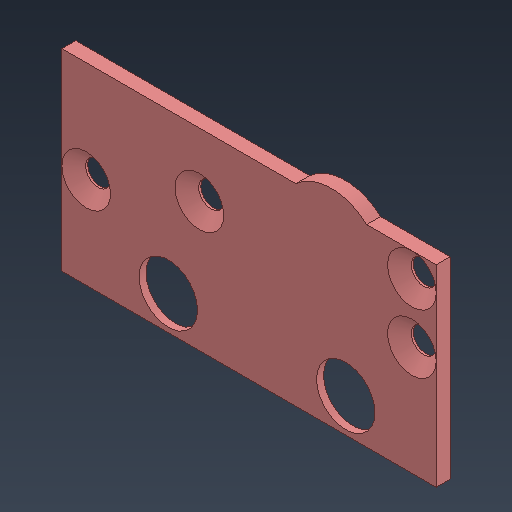
# Autodesk Inventor part: gearbox-holder-wall-right
Saved by Autodesk Inventor 2023 (Build 270158000, 158)
## iProperties
Created: 2025-04-06
Part Number: gearbox-holder-wall-right
Material: ABS Plastic
Document SubType Name: Modeling
Designer: szymo
Density: 1.06 g/cm^3
Appearance: Default(3)
Mass: 2.61652 g
Surface Area: 32.3606 cm^2
Volume: 2.46841 cm^3
Author: szymo
Autodesk Inventor part; units mm, degrees
ref_plane "YZ Plane" through (0, 0, 0) normal (1, 0, 0) x (0, 1, 0)
ref_plane "XZ Plane" through (0, 0, 0) normal (0, 1, 0) x (-1, 0, 0)
ref_plane "XY Plane" through (0, 0, 0) normal (0, 0, 1) x (1, 0, 0)
ref_plane "Work Plane7" through (-17.6, -15.9714, 1.1) normal (0, 0, 1) x (1, 0, 0)
ref_plane "Work Plane10" through (0, 0, 0.1) normal (0, 0, 1) x (1, 0, 0)
sketch "Sketch2" plane through (0, 0, 0.1) normal (0, 0, 1) x (1, 0, 0)
  line L0 (26.9, -14.8376) -> (26.9, 13.5936)
  line L1 (-26.9065, -14.8376) -> (26.9, -14.8376)
  circle A0 centre (-11.6, -9.9714) radius 6 projected
  circle A1 centre (13.9, -9.9714) radius 6 projected
  circle A2 centre (-11.6, -9.9714) radius 6.2
  circle A3 centre (13.9, -9.9714) radius 6.2
  arc A4 (-1.8466, -14.8376) -> (-21.3534, -14.8376) centre (-11.6, -9.9714) ccw
  line L2 (-1.8466, -14.8376) -> (4.1466, -14.8376)
  arc A5 (23.6534, -14.8376) -> (4.1466, -14.8376) centre (13.9, -9.9714) ccw
  line L3 (23.6534, -14.8376) -> (26.9, -14.8376)
  line L4 (26.9, -14.8376) -> (26.9, 12.8624)
  line L5 (26.9, 12.8624) -> (16.8986, 12.8624)
  arc A6 (16.8986, 12.8624) -> (6.7153, 12.8624) centre (11.8069, 7.2876) ccw
  line L6 (6.7153, 12.8624) -> (-26.9, 12.8624)
  line L7 (-26.9, 12.8624) -> (-26.9, -14.8376)
  line L8 (-26.9, -14.8376) -> (-21.3534, -14.8376)
  point P0 (0, 0)
  point P1 (-15.4418, -14.8376)
  point P2 (-7.7582, -14.8376)
  point P3 (10.0582, -14.8376)
  point P4 (17.7418, -14.8376)
  point P5 (-1.8466, -14.8376)
  point P6 (-15.1099, -14.8376)
  point P7 (-8.0901, -14.8376)
  point P8 (-26.9, -14.8376)
  point P9 (26.9, 12.8624)
  dimension "d2" = 0.2
  dimension "d3" = 0.2
  constraints: 18 end point, 6 point on circle, 5 centre point, 1 point on line
  measures "d2" radial gap between concentric circles of A0 A2
  measures "d3" radial gap between concentric circles of A1 A3
extrude "Extrusion2" add sketch "Sketch2" along normal up to surface (1 mm away) contours L1 A5 A4 L7 L6 A6 L5 L0 | L1 A3 A5 | L1 A2 A4
ref_plane "Work Plane6" through (-15.6, -13.9714, 2.1) normal (0, 0, 1) x (1, 0, 0)
ref_plane "Work Plane11" through (0, 0, 1.1) normal (0, 0, 1) x (1, 0, 0)
sketch "Sketch3" plane through (0, 0, 1.1) normal (0, 0, 1) x (1, 0, 0)
  circle A0 centre (-11.6, -9.9714) radius 4 projected
  circle A1 centre (13.9, -9.9714) radius 4 projected
  circle A2 centre (-11.6, -9.9714) radius 4.2
  circle A3 centre (13.9, -9.9714) radius 4.2
  line L0 (-15.7569, -14.8376) -> (-7.4431, -14.8376)
  line L1 (17.7418, -14.8376) -> (23.6534, -14.8376)
  line L2 (9.7431, -14.8376) -> (17.7418, -14.8376)
  line L3 (-15.4418, -14.8376) -> (-26.9, -14.8376) projected
  line L4 (26.9, 12.8624) -> (26.9, -14.8376) projected
  line L5 (16.8986, 12.8624) -> (26.9, 12.8624) projected
  line L6 (-26.9, 12.8624) -> (6.7153, 12.8624) projected
  line L7 (-26.9, -14.8376) -> (-26.9, 12.8624) projected
  arc A4 (-7.7582, -14.8376) -> (-15.4418, -14.8376) centre (-11.6, -9.9714) ccw projected
  line L8 (10.0582, -14.8376) -> (-7.7582, -14.8376) projected
  arc A5 (17.7418, -14.8376) -> (10.0582, -14.8376) centre (13.9, -9.9714) ccw projected
  line L9 (26.9, -14.8376) -> (17.7418, -14.8376) projected
  arc A6 (16.8986, 12.8624) -> (6.7153, 12.8624) centre (11.8069, 7.2876) ccw projected
  point P0 (0, 0)
  point P1 (-15.4418, -14.8376)
  point P2 (-15.4418, -14.8376)
  dimension "d6" = 0.2
  dimension "d7" = 0.2
  constraints: 6 end point, 2 centre point, 1 horizontal
  measures "d6" radial gap between concentric circles of A0 A2
  measures "d7" radial gap between concentric circles of A1 A3
extrude "Extrusion3" add sketch "Sketch3" along normal up to surface (1 mm away) contours L3 L7 L6 A6 L5 L4 L9 L1 A5 L2 L8 L0 A4 | A4 L0 | A5 L2
ref_plane "Work Plane9" through (0, 0, 0) normal (0, 0, -1) x (-1, 0, 0)
sketch "Sketch4" plane through (0, 0, 0) normal (0, 0, -1) x (-1, 0, 0)
  circle A0 centre (-11.8069, 7.2876) radius 1.25 projected
  circle A1 centre (-3.3822, 4.9241) radius 1.25 projected
  circle A2 centre (-1.15, -4.8235) radius 1.25 projected
  circle A3 centre (-11.8069, 7.2876) radius 1.55
  circle A4 centre (-3.3822, 4.9241) radius 1.55
  circle A5 centre (-1.15, -4.8235) radius 1.55
  point P0 (0, 0)
  dimension "d10" = 0.3
  dimension "d11" = 0.3
  dimension "d12" = 0.3
  constraints: 3 centre point
  measures "d10" radial gap between concentric circles of A0 A3
  measures "d11" radial gap between concentric circles of A1 A4
  measures "d12" radial gap between concentric circles of A2 A5
extrude "Extrusion4" cut sketch "Sketch4" against normal blind 1.6 contours A0 | A1 | A2 | A3 | A4 | A5
sketch "Sketch5" plane through (-26.9, -14.8376, 2.1) normal (0, 0, 1) x (1, 0, 0)
  circle A0 centre (15.3, 4.8663) radius 12.5 projected
  line L0 (53.8, 27.7) -> (53.8, 0) projected
  line L1 (43.7986, 27.7) -> (53.8, 27.7) projected
  arc A1 (43.7986, 27.7) -> (33.6153, 27.7) centre (38.7069, 22.1252) ccw projected
  line L2 (0, 27.7) -> (33.6153, 27.7) projected
  line L3 (0, 0) -> (0, 27.7) projected
  line L4 (53.8, 0) -> (0, 0) projected
  circle A2 centre (40.8, 4.8663) radius 4.2 projected
  circle A3 centre (15.3, 4.8663) radius 4.2 projected
  line L5 (0, 27.7) -> (0, 0) projected
  line L6 (0, 19.3663) -> (53.8, 19.3663)
  line L7 (53.8, 0) -> (53.8, 27.7) projected
  line L8 (0, 20.3663) -> (53.8, 20.3663)
  point P0 (26.9, 14.8376)
  point P1 (53.8, 20.3663)
  point P2 (0, 20.3663)
  point P3 (0, 19.3663)
  dimension "d15" = 14.5
  dimension "d16" = 1
  constraints: 4 end point, 4 point on line, 2 perpendicular
  measures "d15" distance from line of L6 A0.centre
  measures "d16" distance between parallel lines of L8 L6
ref_plane "Work Plane12" through (-28.9, -14.8376, 19.8) normal (0, 0, 1) x (1, 0, 0)
extrude "Extrusion5" [suppressed]
sketch "Sketch6" plane through (-26.9, -14.8376, 2.1) normal (0, 0, 1) x (1, 0, 0)
  circle A0 centre (19.7652, 18.5565) radius 2.5 projected
  circle A1 centre (50.3, 24.2) radius 2.5 projected
  circle A2 centre (3.5, 13.1197) radius 2.5 projected
  circle A3 centre (50.3, 15.688) radius 2.5 projected
  line L0 (0, 0) -> (5.5466, 0) projected
  arc A4 (5.5466, 0) -> (25.0534, 0) centre (15.3, 4.8663) ccw projected
  arc A5 (31.0466, 0) -> (50.5534, 0) centre (40.8, 4.8663) ccw projected
  line L1 (50.5534, 0) -> (53.8, 0) projected
  line L2 (53.8, 0) -> (53.8, 27.7) projected
  line L3 (33.6153, 27.7) -> (0, 27.7) projected
  arc A6 (43.7986, 27.7) -> (33.6153, 27.7) centre (38.7069, 22.1252) ccw projected
  line L4 (53.8, 27.7) -> (43.7986, 27.7) projected
  line L5 (0, 27.7) -> (0, 0) projected
  circle A7 centre (38.7069, 22.1252) radius 1.55 projected
  circle A8 centre (30.2822, 19.7618) radius 1.55 projected
  line L6 (25.0534, 0) -> (31.0466, 0) projected
  point P0 (26.9, 14.8376)
  point P1 (3.5, 13.1197)
  point P2 (19.7652, 18.5565)
  point P3 (50.3, 15.688)
  point P4 (50.3, 24.2)
  constraints: 4 coincident
hole "Hole1" at (-23.4, -1.7179, 2.1) at (-7.1348, 3.7189, 2.1) at (23.4, 0.8504, 2.1) at (23.4, 9.3624, 2.1) direction (0, 0, -1) diameter 3.6 depth 3 countersink diameter 7 countersink angle 90 clearance for "Countersunk Flat Head Screw ISO 2009/7046" size "M3" standard "ISO"
ref_plane "Work Plane13" through (-28.9, -14.8376, 19.8) normal (0, 0, 1) x (1, 0, 0)
body "Solid1"
